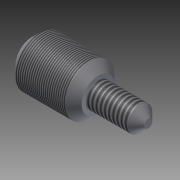
# Autodesk Inventor part: 13_1087_017
Saved by Autodesk Inventor 2014 (Build 180170000, 170)
## iProperties
Created: 2013-09-03
Part Number: 13_1087_017
Material: Allgemein
Document SubType Name: Modeling
Designer: vogel
Density: 1 g/cm^3
Appearance: Vorgabe
Author: vogel
Autodesk Inventor part; units mm, degrees
ref_plane "YZ Plane" through (0, 0, 0) normal (1, 0, 0) x (0, 1, 0)
ref_plane "XZ Plane" through (0, 0, 0) normal (0, 1, 0) x (-1, 0, 0)
ref_plane "XY Plane" through (0, 0, 0) normal (0, 0, 1) x (1, 0, 0)
sketch "Skizze1" plane through (0, 0, 0) normal (0, 0, 1) x (1, 0, 0)
  line L0 (-16.8, 0) -> (2.8, 0) projected
  line L1 (0, -0.6) -> (0, 3.6) projected
  line L2 (0, 1.5) -> (-6, 1.5)
  line L3 (-6, 1.5) -> (-6, 3)
  line L4 (-6, 3) -> (-14, 3)
  line L5 (-14, 3) -> (-14, 0)
  line L6 (-14, 0) -> (0, 0)
  line L7 (0, 0) -> (0, 1.5)
  dimension "d0" = 3
  dimension "d1" = 6
  dimension "d2" = 6
  dimension "d3" = 8
  constraints: 12 end point, 3 perpendicular, 2 collinear, 1 midpoint, 1 parallel, 1 point on line
  measures "d0" diameter of L2 L0
  measures "d1" diameter of L4 L0
  measures "d2" distance of L2.start L2.end
  measures "d3" distance of L3.end L4.end
revolve "Umdrehung1" add sketch "Skizze1" angle 360 about axis through (-10, 0, 0) along (1, 0, 0)
thread "Gewinde1" size "M3x0.5" class "6g" standard "ANSI Metric M Profile" full length
thread "Gewinde2" size "M1x0.25" class "6g" standard "ANSI Metric M Profile" full length
chamfer "Fase1" distance 1 angle 45 3 edges at (-14, -3, 0) (-6, -3, 0) (0, -1.5, 0)
